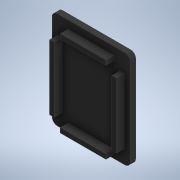
# Autodesk Inventor part: SP19V1 Tapacanto Delantero
Saved by Autodesk Inventor 2021.2 (Build 252289000, 289)
## iProperties
Created: 2026-06-08
Part Number: SP19V1 Tapacanto Delantero
Material: Generic
Document SubType Name: Modeling
Designer: NELSON
Density: 1 g/cm^3
Appearance: Default
Author: NELSON
Autodesk Inventor part; units mm, degrees
ref_plane "YZ Plane" through (0, 0, 0) normal (1, 0, 0) x (0, 1, 0)
ref_plane "XZ Plane" through (0, 0, 0) normal (0, 1, 0) x (-1, 0, 0)
ref_plane "XY Plane" through (0, 0, 0) normal (0, 0, 1) x (1, 0, 0)
sketch "Boceto1" plane through (0, 0, 0) normal (0, 0, 1) x (1, 0, 0)
  line L0 (30, -40) -> (-30, -40)
  line L1 (-30, -40) -> (-30, 40)
  line L2 (-30, 40) -> (30, 40)
  line L3 (30, 40) -> (30, -40)
  line L4 (30, -40) -> (-30, 40) construction
  line L5 (-30, -40) -> (30, 40) construction
  line L6 (33.7, -43.7) -> (-33.7, -43.7)
  line L7 (-33.7, -43.7) -> (-33.7, 43.7)
  line L8 (-33.7, 43.7) -> (33.7, 43.7)
  line L9 (33.7, 43.7) -> (33.7, -43.7)
  line L10 (-33.7, -40) -> (33.7, -40)
  point P0 (0, 0)
  point P1 (30, -40)
  point P2 (-30, -40)
  dimension "d0" = 60
  dimension "d1" = 80
  dimension "d2" = 3.7
  dimension "d20" = 3.7
  constraints: 22 end point, 4 parallel, 3 perpendicular, 2 midpoint, 2 point on line, 1 horizontal, 3 other
  measures "d0" distance of L1.end L2.end
  measures "d1" distance of L0.end L1.end
  measures "d2" distance between parallel lines of L3 L9
  measures "d20" distance between parallel lines of L6 L10
extrude "Extrusión1" add sketch "Boceto1" along normal blind 5 contours L0 L1 L2 L3 | L3 L2 L1 L10 L7 L8 L9
sketch "Boceto2" plane through (0, 0, 5) normal (0, 0, 1) x (1, 0, 0)
  line L0 (29.25, -37.5) -> (-29.25, -37.5)
  line L1 (-29.25, -37.5) -> (-29.25, 37.5)
  line L2 (-29.25, 37.5) -> (29.25, 37.5)
  line L3 (29.25, 37.5) -> (29.25, -37.5)
  line L4 (29.25, -37.5) -> (-29.25, 37.5) construction
  line L5 (-29.25, -37.5) -> (29.25, 37.5) construction
  line L6 (28.75, 37) -> (-28.75, 37)
  line L7 (-28.75, 37) -> (-28.75, -37)
  line L8 (-28.75, -37) -> (28.75, -37)
  line L9 (28.75, -37) -> (28.75, 37)
  line L10 (-24.75, 33) -> (24.75, 33)
  line L11 (24.75, 33) -> (24.75, -33)
  line L12 (24.75, -33) -> (-24.75, -33)
  line L13 (-24.75, -33) -> (-24.75, 33)
  line L14 (19.75, 33) -> (19.75, 37)
  line L15 (-19.75, 33) -> (-19.75, 37)
  line L16 (24.75, 28) -> (28.75, 28)
  line L17 (24.75, -28) -> (28.75, -28)
  line L18 (-24.75, -28) -> (-28.75, -28)
  line L19 (-19.75, -33) -> (-19.75, -37)
  line L20 (19.75, -33) -> (19.75, -37)
  line L21 (-28.75, 28) -> (-24.75, 28)
  point P0 (0, 0)
  dimension "d5" = 58.5
  dimension "d6" = 75
  dimension "d7" = 0.5
  dimension "d8" = 4
  dimension "d9" = 5
  dimension "d10" = 5
  dimension "d11" = 5
  dimension "d12" = 5
  dimension "d13" = 5
  dimension "d14" = 5
  dimension "d15" = 5
  dimension "d16" = 5
  constraints: 44 end point, 16 point on line, 9 perpendicular, 8 parallel, 2 midpoint, 1 horizontal, 6 other
  measures "d5" distance of L1.end L2.end
  measures "d6" distance of L0.end L1.end
  measures "d7" distance between parallel lines of L2 L6
  measures "d8" distance between parallel lines of L6 L10
  measures "d9" distance between parallel lines of L11 L14
  measures "d10" distance between parallel lines of L15 L13
  measures "d11" distance between parallel lines of L16 L10
  measures "d12" distance between parallel lines of L12 L17
  measures "d13" distance between parallel lines of L11 L20
  measures "d14" distance between parallel lines of L13 L19
  measures "d15" distance between parallel lines of L12 L18
  measures "d16" distance between parallel lines of L10 L21
extrude "Extrusión2" add sketch "Boceto2" along normal blind 7 contours L14 L10 L15 L6 | L9 L17 L11 L16 | L21 L13 L18 L7 | L8 L19 L12 L20
fillet "Empalme1" radius 4.716 4 edges at (33.7, 43.7, 2.5) (-33.7, 43.7, 2.5) (33.7, -40, 2.5) (-33.7, -40, 2.5)
chamfer "Chamfer1" distance 0.3 angle 45 8 edges at (0, 43.7, 0) (-32.3187, 42.3187, 0) (-33.7, 1.85, 0) (-32.3187, -38.6187, 0) (0, -40, 0) (32.3187, -38.6187, 0) (33.7, 1.85, 0) (32.3187, 42.3187, 0)
